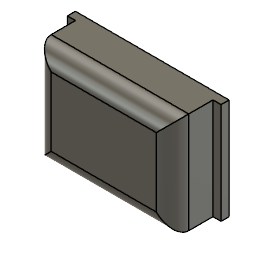
Side-Button (Autodesk Fusion 360 design; units mm, degrees)
Autodesk Fusion 360 part; units mm, degrees
sketch "Sketch1" plane through (0, 0, 0) normal (0, 0, 1) x (1, 0, 0)
  line L0 (-30, 20) -> (-13, 20)
  line L1 (-13, 20) -> (-13, 7.5)
  line L2 (-13, 7.5) -> (-30, 7.5)
  line L3 (-30, 7.5) -> (-30, 20)
  dimension "d1" = 17
  dimension "d2" = 12.5
  constraint horizontal L0
  constraint vertical L1
  constraint horizontal L2
  constraint vertical L3
  measures "d1" distance of L0.start L0.end
  measures "d2" distance of L0.start L2.end
extrude "Extrude1" add sketch "Sketch1" along normal blind 6
fillet "Fillet1" radius 2 4 edges at (-21.5, 20, 6) (-13, 13.75, 6) (-30, 13.75, 6) (-21.5, 7.5, 6)
sketch "Sketch3" plane through (0, 0, 0) normal (0, 0, -1) x (-1, 0, 0)
  line L0 (13, 7.5) -> (30, 7.5)
  line L1 (30, 7.5) -> (30, 20)
  line L2 (30, 20) -> (13, 20)
  line L3 (13, 20) -> (13, 7.5)
  line L4 (13, 20) -> (30, 20)
  line L5 (30, 20) -> (30, 7.5)
  line L6 (30, 7.5) -> (13, 7.5)
  line L7 (13, 7.5) -> (13, 20)
  line L8 (12, 20) -> (31, 20)
  line L9 (12, 7.5) -> (31, 7.5)
  line L10 (12, 20) -> (31, 20)
  line L11 (31, 20) -> (31, 7.5)
  line L12 (31, 7.5) -> (12, 7.5)
  line L13 (12, 7.5) -> (12, 20)
  point P0 (21.5, 20)
  point P1 (21.5, 7.5)
  dimension "d10" = 19
  dimension "d11" = 19
  constraint horizontal L4
  constraint vertical L5
  constraint horizontal L6
  constraint vertical L7
  constraint coincident L0.end L1.start
  constraint coincident L2.end L3.start
  constraint midpoint L8 P0
  constraint coincident L4 P0
  constraint perpendicular L1 L8
  constraint midpoint L9 P1
  constraint coincident L6 P1
  constraint perpendicular L1 L9
  constraint horizontal L10
  constraint vertical L11
  constraint horizontal L12
  constraint vertical L13
  measures "d10" distance of L8.start L8.end
  measures "d11" distance of L9.start L9.end
extrude "Extrude3" add sketch "Sketch3" against normal blind 1 contours L3 L7 L8 L9 L10 L12 L13 | L1 L5 L8 L9 L10 L11 L12
